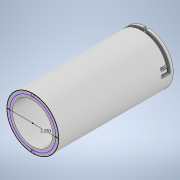
# Autodesk Inventor part: Maze
Saved by Autodesk Inventor 2021 (Build 250183000, 183)
## iProperties
Created: 2020-07-17
Part Number: Maze
Material: Generic
Document SubType Name: Modeling
Designer: saipr
Density: 1 g/cm^3
Appearance: Default
Author: saipr
Autodesk Inventor part; units mm, degrees
ref_plane "YZ Plane" through (0, 0, 0) normal (1, 0, 0) x (0, 1, 0)
ref_plane "XZ Plane" through (0, 0, 0) normal (0, 1, 0) x (-1, 0, 0)
ref_plane "XY Plane" through (0, 0, 0) normal (0, 0, 1) x (1, 0, 0)
sketch "Sketch1" plane through (0, 0, 0) normal (0, 0, 1) x (1, 0, 0)
  circle A0 centre (0, 0) radius 25.4
  circle A1 centre (0, 0) radius 22.225
  line L0 (0, 0) -> (0, 25.4)
  line L1 (0, 0) -> (19.2474, -11.1125)
  line L2 (0, 0) -> (-19.2474, -11.1125)
  line L3 (-19.2474, -11.1125) -> (-21.997, -12.7)
  line L4 (19.2474, -11.1125) -> (21.997, -12.7)
  arc A2 (9.6237, 23.5063) -> (-9.6237, 23.5063) centre (0, 0) ccw
  arc A3 (2.54, 25.2727) -> (-2.54, 25.2727) centre (0, 0) ccw
  arc A4 (21.2995, -13.8381) -> (22.9699, -10.8419) centre (0, 0) ccw
  arc A5 (20.5909, -14.872) -> (23.1385, -10.477) centre (0, 0) ccw
  dimension "d0" = 50.8
  dimension "d1" = 44.45
  dimension "d2" = 120
  dimension "d3" = 120
  dimension "d5" = 25.4
  constraints: 17 point on circle, 10 end point, 5 centre point, 2 coincident, 2 collinear, 1 concentric, 1 vertical, 10 other
  measures "d1" diameter of A1
  measures "d2" angle of L1 L0
  measures "d3" angle of L0 L2
  measures "d5" radius of A2
extrude "Extrusion1" add sketch "Sketch1" along normal blind 127 contours A0 L4 A1 L0 | L0 A1 L3 A0 | A0 L3 A1 L4
sketch "Sketch9" plane through (0, 0, 127) normal (0, 0, 1) x (1, 0, 0)
  circle A0 centre (0, 0) radius 28.575
  circle A1 centre (0, 0) radius 25.4
  circle A2 centre (0, 0) radius 25.4 projected
  arc A3 (1.4111, 25.3608) -> (-1.4111, 25.3608) centre (0, 0) ccw
  line L0 (1.5875, 28.5309) -> (1.4111, 25.3608)
  line L1 (-1.4111, -25.3608) -> (-1.5875, -28.5309)
  line L2 (-1.5875, 28.5309) -> (-1.4111, 25.3608)
  line L3 (1.4111, -25.3608) -> (1.5875, -28.5309)
  point P0 (-1.4111, 25.3608)
  dimension "d62" = 57.15
  constraints: 10 point on circle, 8 end point, 3 centre point, 2 coincident, 1 concentric
  measures "d62" diameter of A0
extrude "Extrusion7" add sketch "Sketch9" against normal blind 127 contours A0 L3 A1 L0 | L2 A1 L1 A0
extrude "Extrusion8" add sketch "Sketch9" against normal blind 120.65 contours L0 A1 L2 A0
ref_plane "Work Plane7" through (0, 0, 6.35) normal (0, 0, -1) x (-1, 0, 0)
sketch "Sketch10" plane through (0, 0, 6.35) normal (0, 0, -1) x (-1, 0, 0)
  circle A0 centre (0, 0) radius 25.4
  circle A1 centre (0, 0) radius 28.575
  line L0 (1.4111, -25.3608) -> (1.5875, -28.5309) projected
  line L1 (0, 0) -> (28.575, 0)
  arc A2 (1.5875, -28.5309) -> (1.5875, 28.5309) centre (0, 0) ccw projected
  line L2 (0, 0) -> (-28.575, 0)
  arc A3 (1.5875, -28.5309) -> (-1.5875, -28.5309) centre (0, 0) ccw projected
  line L3 (1.5875, 28.5309) -> (0, 0)
  line L4 (0, 0) -> (-1.5875, 28.5309)
  point P0 (25.4, 0)
  point P1 (-25.4, 0)
  point P2 (1.4111, 25.3608)
  point P3 (-1.4111, 25.3608)
  constraints: 8 end point, 3 point on circle, 2 coincident, 1 centre point, 1 horizontal, 1 point on line, 2 other
extrude "Extrusion10" cut sketch "Sketch10" along normal blind 3.175 contours A0 L3 A1 L1 | L2 A1 L4 A0
sketch "Sketch11" plane through (0, 0, 6.35) normal (0, 0, -1) x (-1, 0, 0)
  line L0 (-28.575, 0) -> (-25.4, 0) projected
  line L1 (0, 0) -> (-28.575, 0)
  line L2 (-28.575, 0) -> (0, 0)
  arc A0 (28.575, 0) -> (-28.575, 0) centre (0, 0) ccw projected
  line L3 (-28.575, 0) -> (-28.3986, 3.1701)
  arc A1 (-1.5875, 28.5309) -> (-1.5875, -28.5309) centre (0, 0) ccw projected
  line L4 (-28.3986, 3.1701) -> (0, 0)
  line L5 (-28.3986, 3.1701) -> (-27.8716, 6.3011)
  line L6 (-27.8716, 6.3011) -> (-27.0005, 9.3542)
  line L7 (0, 0) -> (-27.8716, 6.3011)
  line L8 (-27.0005, 9.3542) -> (0, 0)
  arc A2 (-1.4111, -25.3608) -> (1.4111, -25.3608) centre (0, 0) ccw projected
  circle A3 centre (0, 0) radius 25.4
  point P0 (-24.7748, 5.6009)
  point P1 (-24.0005, 8.3149)
  point P2 (-25.2432, 2.8179)
  dimension "d77" = 3.175
  dimension "d78" = 3.175
  dimension "d79" = 3.175
  constraints: 16 end point, 3 point on circle, 1 coincident, 1 collinear, 1 horizontal, 3 other
  measures "d77" distance of L0.start L3.end
  measures "d78" distance of L3.end L5.end
  measures "d79" distance of L5.end L6.end
extrude "Extrusion11" cut sketch "Sketch11" against normal blind 6.35 contours L3 L4 A3 L0 | A0 L3 | A0 L6 | L6 L8 A3 L7
body "Solid1"
